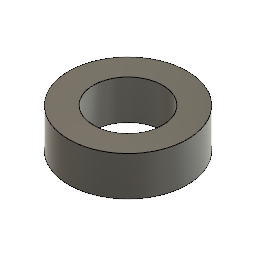
spacer_for_front_axle_2mm (Autodesk Fusion 360 design; units mm, degrees)
Autodesk Fusion 360 part; units mm, degrees
sketch "スケッチ1" plane through (0, 0, 0) normal (0, 1, 0) x (1, 0, 0)
  circle A0 centre (0, 0) radius 1.75
  circle A1 centre (0, 0) radius 3
  dimension "d1" = 3.5
  constraint coincident A0.centre A1.centre
  measures "d1" diameter of A0
extrude "押し出し1" add sketch "スケッチ1" along normal blind 2 makes body 1
copy_body "ボディのコピーと貼り付け1" bodies 1 makes body 2
